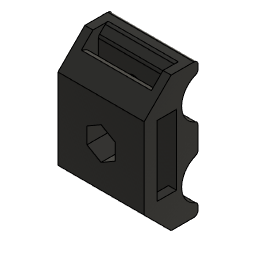
Apollo Yoke Lock B Side [(P)MPLA000000177] v2 (Autodesk Fusion 360 design; units mm, degrees)
Autodesk Fusion 360 part; units mm, degrees
note: some values were not read from the file. Set by a fixed rule: which sketch regions a step uses.
sketch "Sketch1" plane through (0, 0, 0) normal (0, 0, 1) x (1, 0, 0)
  line L0 (16, -4) -> (-16, -4)
  line L1 (-16, -4) -> (-16, 4)
  line L2 (-16, 4) -> (16, 4)
  line L3 (16, 4) -> (16, -4)
  dimension "d1" = 8
  dimension "d2" = 32
  dimension "d20" = 4
  dimension "d21" = 16
  constraint horizontal L0
  constraint vertical L1
  constraint horizontal L2
  constraint vertical L3
  measures "d1" distance of L0.start L2.end
  measures "d2" distance of L1 L3
  measures "d20" distance of origin L2
  measures "d21" distance of origin L1
extrude "Extrude1" add sketch "Sketch1" along normal mid plane 50
sketch "Sketch2" plane through (-16, 0, 0) normal (-1, 0, 0) x (0, 0, 1)
  circle A0 centre (13, 6) radius 8.1
  circle A1 centre (-13, 6) radius 8.1
  line L0 (-25, -4) -> (25, -4)
  line L1 (25, -4) -> (25, 4)
  line L2 (25, 4) -> (-25, 4)
  line L3 (-25, 4) -> (-25, -4)
  dimension "d22" = 16.2
  dimension "d23" = 16.2
  dimension "d24" = 26
  dimension "d25" = 13
  dimension "d70" = 2
  constraint horizontal A0.centre A1.centre
  measures "d22" diameter of A0
  measures "d23" diameter of A1
  measures "d24" horizontal distance of A0.centre A1.centre
  measures "d25" horizontal distance of origin A0.centre
  measures "d70" distance of A0.centre L2
extrude "Extrude2" cut sketch "Sketch2" along normal blind -33 and the other way blind -2 contours A0 L2 | A0 L2 | A1 L2 | A1 L2
sketch "Sketch3" plane through (0, 4, 0) normal (0, 1, 0) x (-1, 0, 0)
  line L0 (-15, -5.1508) -> (15, -5.1508)
  line L1 (15, -5.1508) -> (15, 5.1508)
  line L2 (15, 5.1508) -> (-15, 5.1508)
  line L3 (-15, 5.1508) -> (-15, -5.1508)
  circle A0 centre (0, 0) radius 3
  circle A1 centre (0, 13) radius 3
  circle A2 centre (0, -13) radius 3
  circle A3 centre (0, 13) radius 4
  circle A4 centre (0, -13) radius 4
  line L4 (-16, -5.1508) -> (16, -5.1508)
  line L5 (16, -5.1508) -> (16, 5.1508)
  line L6 (16, 5.1508) -> (-16, 5.1508)
  line L7 (-16, 5.1508) -> (-16, -5.1508)
  dimension "d9" = 6
  dimension "d10" = 6
  dimension "d11" = 6
  dimension "d12" = 8
  dimension "d13" = 8
  dimension "d14" = 26
  dimension "d27" = 13
  constraint coincident A0.centre origin
  constraint concentric A1 A3
  constraint concentric A2 A4
  constraint vertical A0.centre A1.centre
  constraint vertical A0.centre A2.centre
  measures "d9" diameter of A0
  measures "d10" diameter of A1
  measures "d11" diameter of A2
  measures "d12" diameter of A3
  measures "d13" diameter of A4
  measures "d14" distance of A1.centre A2.centre
  measures "d27" distance of A0.centre A1.centre
extrude "Extrude3" cut sketch "Sketch3" against normal blind 13 contours A0 | A1 | A2
sketch "Sketch4" plane through (0, -4, 0) normal (0, -1, 0) x (1, 0, 0)
  circle A0 centre (0, -13) radius 3
  circle A1 centre (0, 0) radius 3
  circle A2 centre (0, 13) radius 3
  circle A3 centre (0, 13) radius 3
  circle A4 centre (0, 0) radius 3
  circle A5 centre (0, -13) radius 3
  line L0 (-16, 25) -> (-16, -25)
  line L1 (16, -25) -> (16, 25)
  line L2 (-19, 25) -> (19, 25)
  line L3 (19, 25) -> (19, -25)
  line L4 (19, -25) -> (-19, -25)
  line L5 (-19, -25) -> (-19, 25)
  line L6 (-13, 25) -> (13, 25)
  line L7 (13, 25) -> (13, -25)
  line L8 (13, -25) -> (-13, -25)
  line L9 (-13, -25) -> (-13, 25)
  line L10 (-19, 13) -> (19, 13)
  line L11 (19, 13) -> (19, -13)
  line L12 (19, -13) -> (-19, -13)
  line L13 (-19, -13) -> (-19, 13)
  line L14 (16, 25) -> (-16, 25)
  line L15 (-16, -25) -> (16, -25)
  dimension "d44" = 3
  dimension "d45" = 3
  dimension "d46" = 26
  dimension "d47" = 13
  dimension "d48" = 26
  dimension "d49" = 13
  constraint horizontal L2
  constraint vertical L3
  constraint horizontal L4
  constraint vertical L5
  constraint horizontal L6
  constraint vertical L7
  constraint horizontal L8
  constraint vertical L9
  constraint coincident L4 L7.end
  constraint coincident L2 L6.start
  constraint horizontal L10
  constraint vertical L11
  constraint horizontal L12
  constraint vertical L13
  constraint coincident L3 L11.end
  constraint coincident L5 L10.start
  constraint collinear L6 L14
  constraint collinear L4 L15
  measures "d44" distance of L0 L5
  measures "d45" distance of L1 L3
  measures "d46" distance of L7 L9
  measures "d47" distance of A1.centre L7
  measures "d48" distance of L10 L12
  measures "d49" distance of A1.centre L10
extrude "Extrude5" add sketch "Sketch4" along normal blind 7 contours L1 L4 L7 L12 L15 | L0 L4 L9 L12 L15 | L1 L2 L7 L10 L14 | L0 L2 L9 L10 L14
extrude "Extrude4" cut sketch "Sketch3" against normal blind 7 contours A3 | A4
chamfer "Chamfer5" distance 3 angle 45 2 edges at (0, -4, -25) (0, -4, 25)
fillet "Fillet1" radius 1.5 10 edges at (0, 4, 25) (0, 4, -25) (0, 4, -20.8492) (0, 4, -5.1508) (0, 4, 5.1508) (0, 4, 20.8492) (0, -1, 25) (0, -4, 22) (0, -4, -22) (0, -1, -25)
sketch "Sketch6" plane through (0, -11, 0) normal (0, -1, 0) x (1, 0, 0)
  line L0 (16, 25) -> (13, 25)
  line L1 (13, 25) -> (13, 13)
  line L2 (13, 13) -> (16, 13)
  line L3 (16, 13) -> (16, 25)
  line L4 (16, 25) -> (-16, 25)
  line L5 (-16, 25) -> (-16, -25)
  line L6 (-16, -25) -> (16, -25)
  line L7 (16, -25) -> (16, 25)
  point P0 (-16, -25)
  constraint horizontal L4
  constraint vertical L5
  constraint horizontal L6
  constraint vertical L7
  constraint coincident L0.start L3.end
  constraint coincident P0 L5.end
extrude "Extrude8" add sketch "Sketch6" along normal blind 5
extrude "Extrude9" add 1 faces at (-4.3333, -11, 4.3333) along direction (0, 1, 0) blind 2.8
chamfer "Chamfer7" distance 10 angle 45 2 edges at (0, -16, 25) (0, -16, -25)
chamfer "Chamfer6" distance 3 angle 45 4 edges at (16, -8.2, 0) (-16, -8.2, 0) (0, -8.2, -22.8) (0, -8.2, 22.8)
sketch "Sketch7" plane through (0, -16, 0) normal (0, -1, 0) x (1, 0, 0)
  line L0 (-16, -15) -> (16, -15)
  line L1 (16, -15) -> (16, 15)
  line L2 (16, 15) -> (-16, 15)
  line L3 (-16, 15) -> (-16, -15)
  line L4 (5.25, 3.0311) -> (0, 6.0622)
  line L5 (0, 6.0622) -> (-5.25, 3.0311)
  line L6 (-5.25, 3.0311) -> (-5.25, -3.0311)
  line L7 (-5.25, -3.0311) -> (0, -6.0622)
  line L8 (0, -6.0622) -> (5.25, -3.0311)
  line L9 (5.25, -3.0311) -> (5.25, 3.0311)
  dimension "d66" = 5.25
  measures "d66" distance of origin L9
extrude "Extrude10" cut sketch "Sketch7" against normal blind 8 contours L4 L5 L6 L7 L8 L9
chamfer "Chamfer8" [suppressed]
equation "d3 = d216 / 2"
equation "d17 = d241 / 2"
equation "d20 = d1 / 2"
equation "d21 = d2 / 2"
equation "d25 = d24 / 2"
equation "d27 = d14 / 2"
equation "d47 = d46 / 2"
equation "d49 = d48 / 2"
